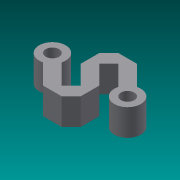
# Autodesk Inventor part: Sawaiz Logo Ribbon 2
Saved by Autodesk Inventor 2015 (Build 190159000, 159)
## iProperties
Created: 2015-06-22
Part Number: Sawaiz Logo Ribbon 2
Material: Generic
Document SubType Name: Modeling
Designer: Sawaiz Syed
Density: 1 g/cm^3
Appearance: Default
Author: Sawaiz Syed
Autodesk Inventor part; units mm, degrees
ref_plane "YZ Plane" through (0, 0, 0) normal (1, 0, 0) x (0, 1, 0)
ref_plane "XZ Plane" through (0, 0, 0) normal (0, 1, 0) x (-1, 0, 0)
ref_plane "XY Plane" through (0, 0, 0) normal (0, 0, 1) x (1, 0, 0)
sketch "Sketch1" plane through (0, 0, 0) normal (0, 0, 1) x (1, 0, 0)
  circle A0 centre (0, 0) radius 2.5
  circle A1 centre (0, 0) radius 5
  line L0 (-1.7678, -1.7678) -> (-12.3744, 8.8388)
  line L1 (-12.3744, 8.8388) -> (-15.9099, 5.3033)
  line L2 (-15.9099, 5.3033) -> (-8.8388, -1.7678)
  line L3 (-8.8388, -1.7678) -> (-8.8388, -8.8388)
  line L4 (-8.8388, -8.8388) -> (-12.3744, -12.3744)
  line L5 (-19.4454, -12.3744) -> (-30.052, -1.7678)
  line L6 (1.7678, 1.7678) -> (-8.8388, 12.3744)
  line L7 (-15.9099, 12.3744) -> (-19.4454, 8.8388)
  line L8 (-19.4454, 8.8388) -> (-19.4454, 1.7678)
  line L9 (-19.4454, 1.7678) -> (-12.3744, -5.3033)
  line L10 (-12.3744, -5.3033) -> (-15.9099, -8.8388)
  line L11 (-15.9099, -8.8388) -> (-26.5165, 1.7678)
  line L12 (-26.5165, 1.7678) -> (-30.052, -1.7678)
  line L13 (-1.7678, -1.7678) -> (1.7678, 1.7678)
  circle A2 centre (-28.2843, 0) radius 2.5
  circle A3 centre (-28.2843, 0) radius 5
  line L14 (-15.9099, 12.3744) -> (-8.8388, 12.3744)
  line L15 (-19.4454, -12.3744) -> (-12.3744, -12.3744)
  dimension "d0" = 5
  dimension "d1" = 10
  dimension "d3" = 90
  dimension "d6" = 135
  dimension "d7" = 135
  dimension "d8" = 90
  dimension "d9" = 5
  dimension "d12" = 10
  dimension "d13" = 15
  dimension "d14" = 15
  dimension "d31" = 7.0711
  dimension "d32" = 15
  dimension "d33" = 7.0711
  dimension "d34" = 15
  dimension "d35" = 7.0711
  dimension "d36" = 7.0711
  dimension "d37" = 5
  dimension "d38" = 90
  dimension "d39" = 135
  dimension "d40" = 5
  dimension "d41" = 5
  constraints: 32 end point, 4 centre point, 4 parallel, 3 coincident, 3 tangent, 2 horizontal, 2 perpendicular, 2 point on circle, 1 collinear, 1 midpoint, 1 vertical
  measures "d0" diameter of A0
  measures "d1" diameter of A1
  measures "d3" angle of L1 L0
  measures "d6" angle of L2 L3
  measures "d7" angle of L3 L4
  measures "d8" angle of L4 L5
  measures "d9" distance of L11.end L5.end
  measures "d12" diameter of A3
  measures "d13" distance of L0.start L0.end
  measures "d14" distance of L10.end L11.end
  measures "d31" distance of L7.start L6.end
  measures "d32" distance of L6.start L6.end
  measures "d33" distance of L5.start L4.end
  measures "d34" distance of L5.start L5.end
  measures "d35" distance of L7.end L8.end
  measures "d36" distance of L2.end L3.end
  measures "d37" distance between parallel lines of L9 L2
  measures "d38" angle of L2 L1
  measures "d39" angle of L8 L7
  measures "d40" distance of L0.end L1.end
  measures "d41" distance of L9.end L10.end
extrude "Extrusion6" add sketch "Sketch1" along normal blind 10 contours A0 L6 A1 L0 | A0 L0 A1 L6 | A1 L0 L1 L2 L3 L4 L15 L5 A3 L11 L10 L9 L8 L7 L14 L6 | A3 L5 A2 L11 | L11 A2 L5 A3 | A2 L12 picked at (-27.7945, -0.6742)
sketch "Sketch4" plane through (0, 0, 10) normal (0, 0, 1) x (1, 0, 0)
  line L0 (-1.2941, 4.8296) -> (-8.8388, 12.3744) projected
  line L1 (-8.8388, 12.3744) -> (-15.9099, 12.3744) projected
  line L2 (-15.9099, 12.3744) -> (-19.4454, 8.8388) projected
  line L3 (-19.4454, 8.8388) -> (-19.4454, 1.7678) projected
  line L4 (-19.4454, 1.7678) -> (-12.3744, -5.3033) projected
  line L5 (-12.3744, -5.3033) -> (-15.9099, -8.8388) projected
  line L6 (-15.9099, -8.8388) -> (-23.4546, -1.2941) projected
  arc A0 (-23.4546, -1.2941) -> (-26.9902, -4.8296) centre (-28.2843, 0) ccw projected
  line L7 (-26.9902, -4.8296) -> (-19.4454, -12.3744) projected
  line L8 (-19.4454, -12.3744) -> (-12.3744, -12.3744) projected
  line L9 (-12.3744, -12.3744) -> (-8.8388, -8.8388) projected
  line L10 (-8.8388, -8.8388) -> (-8.8388, -1.7678) projected
  line L11 (-8.8388, -1.7678) -> (-15.9099, 5.3033) projected
  line L12 (-15.9099, 5.3033) -> (-12.3744, 8.8388) projected
  line L13 (-12.3744, 8.8388) -> (-4.8296, 1.2941) projected
  arc A1 (-4.8296, 1.2941) -> (-1.2941, 4.8296) centre (0, 0) ccw projected
  line L14 (-30.052, -1.7678) -> (-26.5165, 1.7678) projected
  arc A2 (-26.5165, 1.7678) -> (-30.052, -1.7678) centre (-28.2843, 0) ccw projected
  circle A3 centre (0, 0) radius 2.5 projected
  circle A4 centre (-28.2843, 0) radius 2.5
  constraints: 1 centre point, 1 coincident, 1 concentric
extrude "Extrusion7" cut sketch "Sketch4" against normal blind 10 contours L14 A4
equation "\"d1\" = 2 * d0"
equation "\"d9\" = d0"
equation "\"d12\" = d1"
equation "\"d13\" = 3 * d0"
equation "\"d14\" = d13"
body "Solid4"
